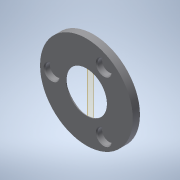
# Autodesk Inventor part: 02_SMLM_Holdre_Bottom
Saved by Autodesk Inventor 2022 (Build 260153000, 153)
## iProperties
Created: 2021-11-24
Part Number: 02_SMLM_Holdre_Bottom
Material: Generisch
Document SubType Name: Modeling
Designer: Muriel
Density: 1 g/cm^3
Appearance: Vorgabe
Author: Muriel
Autodesk Inventor part; units mm, degrees
ref_plane "YZ Plane" through (0, 0, 0) normal (1, 0, 0) x (0, 1, 0)
ref_plane "XZ Plane" through (0, 0, 0) normal (0, 1, 0) x (-1, 0, 0)
ref_plane "XY Plane" through (0, 0, 0) normal (0, 0, 1) x (1, 0, 0)
ref_plane "Arbeitsebene1" through (0, -18.5, -1.048) normal (1, 0, 0) x (0, 0, -1)
sketch "Skizze1" plane through (0, -18.5, -1.048) normal (1, 0, 0) x (0, 0, -1)
  line L0 (-1.65, 12.5) -> (-1.5, 12.5)
  line L1 (-1.5, -12.5) -> (-1.5, 12.5) projected
  line L2 (-1.65, 12.5) -> (-1.65, -12.5) projected
  line L3 (8.4324, 0) -> (-3.3304, 0)
  line L4 (-1.6429, 13.1) -> (-1.65, 13.1)
  line L5 (-1.65, 13.1) -> (-1.65, 11.5)
  line L6 (-1.65, 11.5) -> (-2.05, 11.5)
  line L7 (-2.05, 11.5) -> (-2.05, 23.9922)
  line L8 (-2.05, 23.9922) -> (1.05, 23.9922)
  line L9 (1.05, 23.9922) -> (1.05, 14.9922)
  line L10 (1.552, 13.5) -> (-1.048, 13.5) construction
  line L11 (-1.65, 13.1) -> (-1.4, 13.1)
  line L12 (-1.4, 13.1) -> (-1.4, 14.9922)
  line L13 (-1.4, 14.9922) -> (1.05, 14.9922)
  point P0 (-1.048, 18.5)
  dimension "d0" = 0.4
  dimension "d1" = 3.1
  dimension "d2" = 9
  dimension "d3" = 0.6
  dimension "d4" = 0
  dimension "d5" = 1
  dimension "d6" = 0.25
  constraints: 24 end point, 6 perpendicular, 5 horizontal, 1 collinear, 6 other
  measures "d0" distance of L5.end L6.end
  measures "d1" distance of L7.end L8.end
  measures "d2" distance of L8.end L9.end
  measures "d3" distance from line of L0 L4.start
  measures "d4" distance between parallel lines of L2 L5
  measures "d5" distance between parallel lines of L0 L6
  measures "d6" distance between parallel lines of L12 L5
revolve "Umdrehung1" add sketch "Skizze1" angle 360 about axis through (0, -18.5, -9.4804) along (0, 0, 1) contours L2 L6 L7 L8 L9 L13 L12 L11 L4 L5
sketch "Skizze2" plane through (0, -18.5, 1.002) normal (0, 0, -1) x (-1, 0, 0)
  circle A0 centre (0, 0) radius 14.9922 projected
  circle A1 centre (0, 0) radius 23.9922 projected
  line L0 (19.4922, 0) -> (-9.7461, -16.8807) construction
  line L1 (-9.7461, -16.8807) -> (-9.7461, 16.8807) construction
  line L2 (-9.7461, 16.8807) -> (19.4922, 0) construction
  circle A2 centre (19.4922, 0) radius 4
  circle A3 centre (-9.7461, -16.8807) radius 4
  circle A4 centre (-9.7461, 16.8807) radius 4
  point P0 (0, 18.5)
  dimension "d8" = 47.9844
  dimension "d9" = 29.9844
  dimension "d10" = 19.4922
  dimension "d11" = 8
  dimension "d12" = 8
  dimension "d13" = 8
  constraints: 6 end point, 4 coincident, 3 centre point, 7 other
  measures "d8" diameter of A1
  measures "d9" diameter of A0
  measures "d10" distance of L0.start A0.centre
  measures "d11" diameter of A2
  measures "d12" diameter of A3
  measures "d13" diameter of A4
extrude "Extrusion1" cut sketch "Skizze2" along normal blind 3 contours A2 | A3 | A4
chamfer "Fase1" distance 0.5 angle 45 3 edges at (13.7461, -1.6193, 1.002) (13.7461, -35.3807, 1.002) (-15.4922, -18.5, 1.002)
sketch "Skizze3" plane through (0, -18.5, 1.002) normal (0, 0, 1) x (1, 0, 0)
  arc A0 (11.9961, -20.7778) -> (11.9961, 20.7778) centre (0, 0) ccw projected
  circle A1 centre (0, 0) radius 23.9922
  circle A2 centre (0, 0) radius 26
  point P0 (0, 18.5)
  point P1 (11.9961, -20.7778)
  point P2 (11.9961, 20.7778)
  dimension "d19" = 52
  constraints: 2 centre point, 2 coincident, 1 concentric
  measures "d19" diameter of A2
extrude "Extrusion2" add sketch "Skizze3" against normal blind 4
chamfer "Fase2" distance 0.6 angle 45 1 edges at (-11.9961, -39.2778, -2.998)
equation "\"d10\" = 0.25 * d9 + 0.25 * d8"
